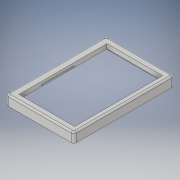
# Autodesk Inventor part: top lcd mount
Saved by Autodesk Inventor 2019.3 (Build 233278000, 278)
## iProperties
Created: 2020-01-08
Part Number: top lcd mount
Material: Generic
Document SubType Name: Modeling
Designer: Emile
Density: 1 g/cm^3
Appearance: Default
Author: Emile
Autodesk Inventor part; units mm, degrees
ref_plane "YZ Plane" through (0, 0, 0) normal (1, 0, 0) x (0, 1, 0)
ref_plane "XZ Plane" through (0, 0, 0) normal (0, 1, 0) x (-1, 0, 0)
ref_plane "XY Plane" through (0, 0, 0) normal (0, 0, 1) x (1, 0, 0)
sketch "Sketch1" plane through (0, 0, 0) normal (0, 1, 0) x (-1, 0, 0)
  line L0 (-76.3737, 106.9555) -> (27.9763, 106.9555)
  line L1 (27.9763, 106.9555) -> (27.9763, -58.1445)
  line L2 (27.9763, -58.1445) -> (-76.3737, -58.1445)
  line L3 (-76.3737, -58.1445) -> (-76.3737, 106.9555)
  line L4 (-76.3737, 106.9555) -> (27.9763, -58.1445) construction
  line L5 (27.9763, 106.9555) -> (-76.3737, -58.1445) construction
  line L6 (38.2263, 114.9555) -> (38.2263, -66.9445)
  line L7 (38.2263, -66.9445) -> (-82.8737, -66.9445)
  line L8 (-82.8737, -66.9445) -> (-82.8737, 114.9555)
  line L9 (-82.8737, 114.9555) -> (38.2263, 114.9555)
  line L10 (41.2263, -69.9445) -> (41.2263, 117.9555)
  line L11 (41.2263, 117.9555) -> (-85.8737, 117.9555)
  line L12 (-85.8737, 117.9555) -> (-85.8737, -69.9445)
  line L13 (-85.8737, -69.9445) -> (41.2263, -69.9445)
  point P0 (-24.1987, 24.4055)
  dimension "d17" = 104.35
  dimension "d18" = 165.1
  dimension "d19" = 8.8
  dimension "d20" = 6.5
  dimension "d21" = 8
  dimension "d22" = 10.25
  dimension "d23" = 3
  constraints: 28 end point, 7 perpendicular, 2 midpoint, 2 parallel, 1 horizontal, 1 vertical, 3 other
  measures "d17" distance of L1.end L2.end
  measures "d18" distance of L0.end L1.end
  measures "d19" distance between parallel lines of L2 L7
  measures "d20" distance between parallel lines of L3 L8
  measures "d21" distance between parallel lines of L0 L9
  measures "d22" distance between parallel lines of L1 L6
  measures "d23" distance between parallel lines of L6 L10
extrude "Extrusion1" add sketch "Sketch1" along normal blind 8.4 contours L6 L7 L8 L9 | L13 L12 L11 L10
extrude "Extrusion3" add sketch "Sketch1" against normal blind 10 contours L13 L12 L11 L10
fillet "Fillet3" radius 5 4 edges at (-41.2263, -0.8, 117.9555) (-41.2263, -0.8, -69.9445) (85.8737, -0.8, 117.9555) (85.8737, -0.8, -69.9445)
fillet "Fillet4" radius 3 8 edges at (22.3237, 8.4, -69.9445) (-39.7619, 8.4, -68.48) (-41.2263, 8.4, 24.0055) (-39.7619, 8.4, 116.491) (22.3237, 8.4, 117.9555) (84.4092, 8.4, 116.491) (85.8737, 8.4, 24.0055) (84.4092, 8.4, -68.48)
sketch "Sketch4" plane through (0, 0, 0) normal (0, -1, 0) x (1, 0, 0)
  line L0 (-38.2263, 112.9555) -> (-38.2263, -64.9445) projected
  line L1 (-27.9763, 106.9555) -> (-27.9763, -58.1445) projected
  line L2 (-38.2263, 64.9555) -> (-27.9763, 64.9555)
  line L3 (-27.9763, 64.9555) -> (-27.9763, 2.9555)
  line L4 (-27.9763, 2.9555) -> (-38.2263, 2.9555)
  line L5 (-38.2263, 2.9555) -> (-38.2263, 64.9555)
  line L6 (-38.2263, 114.9555) -> (82.8737, 114.9555) projected
  point P0 (0, 0)
  dimension "d28" = 50
  dimension "d29" = 62
  constraints: 8 end point, 2 parallel, 2 point on line, 1 horizontal, 1 perpendicular
  measures "d28" distance between parallel lines of L6 L2
  measures "d29" distance between parallel lines of L4 L2
extrude "Extrusion4" cut sketch "Sketch4" against normal blind 3.5
body "Solid1"
